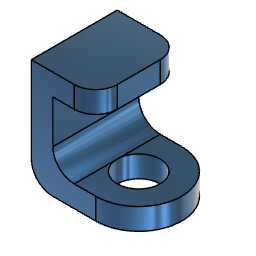
Ex3 (Autodesk Fusion 360 design; units mm, degrees)
Autodesk Fusion 360 part; units mm, degrees
note: some values were not read from the file. Chosen so that the rebuilt part matches the saved one: which face or edge a step refers to.
sketch "Sketch1" plane through (0, 0, 0) normal (0, 0, 1) x (1, 0, 0)
  line L0 (0, 0) -> (20, 0)
  line L1 (20, 40) -> (0, 40)
  line L2 (0, 40) -> (0, 0)
  arc A0 (20, 0) -> (20, 40) centre (20, 20) ccw
  circle A1 centre (20, 20) radius 10
  dimension "d1" = 20
  dimension "d2" = 40
  dimension "d3" = 20
  constraint horizontal L0
  constraint horizontal L1
  constraint vertical L2
  constraint coincident L0.start L2.end
  constraint concentric A0 A1
  measures "d1" distance of L0.start L0.end
  measures "d2" distance of L0.start L1.end
  measures "d3" diameter of A1
extrude "Extrude1" add sketch "Sketch1" along normal blind 10
sketch "Sketch2" plane through (0, 0, 0) normal (-1, 0, 0) x (0, -1, 0)
  line L0 (-40, 0) -> (0, 0)
  line L1 (0, 0) -> (0, 10)
  line L2 (0, 10) -> (-40, 10)
  line L3 (-40, 10) -> (-40, 0)
  line L4 (0, 0) -> (-40, 0)
  line L5 (-40, 0) -> (-40, 40.06)
  line L6 (-40, 40.06) -> (0, 40.06)
  line L7 (0, 40.06) -> (0, 0)
  dimension "d6" = 40
  dimension "d7" = 40.06
  constraint horizontal L4
  constraint vertical L5
  constraint horizontal L6
  constraint vertical L7
  constraint coincident L0.end L1.start
  measures "d6" distance of L0.end L0.start
  measures "d7" distance of L0.end L6.end
extrude "Extrude2" add sketch "Sketch2" along normal blind 10
sketch "Sketch3" plane through (0, 0, 40.06) normal (0, 0, 1) x (-1, 0, 0)
  line L0 (0, 0) -> (0, -40)
  line L1 (0, -40) -> (10, -40)
  line L2 (10, -40) -> (10, 0)
  line L3 (10, 0) -> (0, 0)
  line L4 (10, 0) -> (-20, 0)
  line L5 (-20, 0) -> (-20, -40)
  line L6 (-20, -40) -> (10, -40)
  line L7 (10, -40) -> (10, 0)
  dimension "d10" = 30
  constraint horizontal L4
  constraint vertical L5
  constraint horizontal L6
  constraint vertical L7
  constraint coincident L2.end L3.start
  measures "d10" distance of L2.end L4.end
extrude "Extrude3" add sketch "Sketch3" along normal blind 10
fillet "Fillet1" radius 10 1 edges at (0, 20, 10)
fillet "Fillet2" radius 10 1 edges at (-10, 20, 0)
fillet "Fillet3" radius 10 2 edges at (20, 0, 45.06) (20, 40, 45.06)
